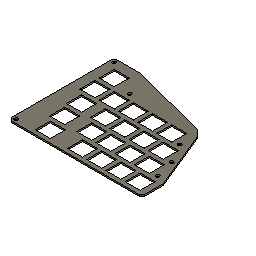
Main Board Plate v2 (Autodesk Fusion 360 design; units mm, degrees)
Autodesk Fusion 360 part; units mm, degrees
note: some values were not read from the file. Set by a fixed rule: which sketch regions a step uses.
(part 1 of 2)
sketch "Sketch1" plane through (0, 0, 0) normal (0, 1, 0) x (1, 0, 0)
  line L0 (0, 0) -> (124, 0)
  line L1 (124, 0) -> (124, 165.5)
  line L2 (124, 165.5) -> (0, 165.5)
  line L3 (0, 165.5) -> (0, 0)
  dimension "d1" = 124
  dimension "d2" = 165.5
  constraint horizontal L0
  constraint vertical L1
  constraint horizontal L2
  constraint vertical L3
  constraint coincident L0.start L3.end
  measures "d1" distance of L0.start L0.end
  measures "d2" distance of L0.start L2.end
extrude "Extrude1" add sketch "Sketch1" along normal blind 1.4
sketch "Sketch2" plane through (0, 1.4, 0) normal (0, 1, 0) x (-1, 0, 0)
  line L0 (0, -165.5) -> (0, 0)
  line L1 (0, 0) -> (-124, 0)
  line L2 (-124, 0) -> (-124, -165.5)
  line L3 (-124, -165.5) -> (0, -165.5)
  line L4 (0, 0) -> (-2.5, 0)
  line L5 (0, 0) -> (0, -2.5)
  line L6 (0, -2.5) -> (-2.5, 0)
  line L7 (-124, 0) -> (-124, -2.5)
  line L8 (-124, 0) -> (-121.5, 0)
  line L9 (-121.5, 0) -> (-124, -2.5)
  line L10 (0, -165.5) -> (0, -163)
  line L11 (0, -165.5) -> (-2.5, -165.5)
  line L12 (-2.5, -165.5) -> (0, -163)
  dimension "d5" = 2.5
  dimension "d6" = 2.5
  dimension "d7" = 2.5
  dimension "d8" = 2.5
  dimension "d9" = 2.5
  constraint coincident L0.end L1.start
  constraint perpendicular L0 L4
  constraint perpendicular L1 L5
  constraint coincident L1.end L2.start
  constraint perpendicular L1 L7
  constraint perpendicular L7 L8
  constraint coincident L0.start L3.end
  constraint coincident L0 L10.end
  constraint perpendicular L1 L10
  constraint perpendicular L10 L11
  measures "d5" distance of L0.end L4.end
  measures "d6" distance of L0.end L5.end
  measures "d7" distance of L1.end L7.end
  measures "d8" distance of L1.end L8.end
  measures "d9" distance of L0.start L11.end
extrude "Extrude2" cut sketch "Sketch2" against normal blind 2 contours L0 L3 L10 L11 L12 | L0 L1 L4 L5 L6 | L1 L2 L7 L8 L9
sketch "Sketch3" plane through (0, 1.4, 0) normal (0, 1, 0) x (-1, 0, 0)
  line L0 (0, -2.5) -> (-2.5, 0)
  line L1 (-2.5, 0) -> (-121.5, 0)
  line L2 (-121.5, 0) -> (-124, -2.5)
  line L3 (-124, -2.5) -> (-124, -165.5)
  line L4 (-124, -165.5) -> (-2.5, -165.5)
  line L5 (-2.5, -165.5) -> (0, -163)
  line L6 (0, -163) -> (0, -2.5)
  line L7 (-2.5, -165.5) -> (0, -165.5)
  line L8 (0, -165.5) -> (-25, -165.5)
  line L9 (0, 0) -> (-96.5, 0)
  line L10 (-96.5, 0) -> (-96.5, -117.5)
  line L11 (0, 0) -> (-102, 0)
  line L12 (-102, 0) -> (-102, -112)
  line L13 (-124, 0) -> (-124, -58)
  line L14 (-25, -165.5) -> (-96.5, -117.5)
  line L15 (-96.5, -117.5) -> (-102, -112)
  line L16 (-102, -112) -> (-124, -58)
  line L17 (-124, -58) -> (-124, -165.5)
  line L18 (-124, -165.5) -> (-25, -165.5)
  dimension "d12" = 25
  dimension "d13" = 96.5
  dimension "d14" = 117.5
  dimension "d15" = 102
  dimension "d16" = 112
  dimension "d17" = 58
  constraint coincident L4.end L5.start
  constraint parallel L4 L7
  constraint parallel L4 L8
  constraint coincident L9.start L11.start
  constraint parallel L1 L9
  constraint perpendicular L1 L10
  constraint parallel L9 L11
  constraint perpendicular L11 L12
  constraint vertical L13
  constraint coincident L3.end L4.start
  measures "d12" distance of L7.end L8.end
  measures "d13" distance of L9.start L9.end
  measures "d14" distance of L9.end L10.end
  measures "d15" distance of L9.start L11.end
  measures "d16" distance of L11.end L12.end
  measures "d17" distance of L13.start L13.end
extrude "Extrude3" cut sketch "Sketch3" against normal blind 5 contours L3 L4 L14 L15 L16 L17 L18
sketch "Sketch4" plane through (0, 1.4, 0) normal (0, 1, 0) x (-1, 0, 0)
  line L0 (-124, -58) -> (-102, -112)
  line L1 (-102, -112) -> (-96.5, -117.5)
  line L2 (-96.5, -117.5) -> (-25, -165.5)
  line L3 (-25, -165.5) -> (-2.5, -165.5)
  line L4 (-2.5, -165.5) -> (0, -163)
  line L5 (0, -163) -> (0, -2.5)
  line L6 (0, -2.5) -> (-2.5, 0)
  line L7 (-2.5, 0) -> (-121.5, 0)
  line L8 (-121.5, 0) -> (-124, -2.5)
  line L9 (-124, -2.5) -> (-124, -58)
  line L10 (0, 0) -> (0, -136.5)
  line L11 (0, -136.5) -> (-30, -136.5)
  line L12 (-25, -165.5) -> (-25, -136.5)
  line L13 (-25, -136.5) -> (-96.5, -117.5)
  dimension "d20" = 136.5
  constraint coincident L10.start origin
  constraint parallel L5 L10
  constraint perpendicular L5 L11
  constraint coincident L2.end L3.start
  constraint coincident L11 L12.end
  constraint perpendicular L11 L12
  constraint coincident L1.end L2.start
  measures "d20" distance of L10.start L10.end
extrude "Extrude4" cut sketch "Sketch4" against normal blind 5 contours L2 L12 L13 | L3 L4 L5 L11 L12
sketch "Sketch5" plane through (0, 1.4, 0) normal (0, 1, 0) x (-1, 0, 0)
  line L0 (-25, -136.5) -> (0, -136.5)
  line L1 (0, -136.5) -> (0, -2.5)
  line L2 (0, -2.5) -> (-2.5, 0)
  line L3 (-2.5, 0) -> (-121.5, 0)
  line L4 (-121.5, 0) -> (-124, -2.5)
  line L5 (-124, -2.5) -> (-124, -58)
  line L6 (-124, -58) -> (-102, -112)
  line L7 (-102, -112) -> (-96.5, -117.5)
  line L8 (-96.5, -117.5) -> (-25, -136.5)
  line L9 (0, -136.5) -> (0, -134)
  line L10 (0, -136.5) -> (-2.5, -136.5)
  line L11 (-2.5, -136.5) -> (0, -134)
  dimension "d23" = 2.5
  constraint coincident L0.end L1.start
  constraint coincident L1 L9.end
  constraint perpendicular L0 L9
  constraint perpendicular L9 L10
  measures "d23" distance of L0.end L10.end
extrude "Extrude5" cut sketch "Sketch5" against normal blind 5 contours L0 L1 L9 L10 L11
sketch "Sketch6" plane through (0, 1.4, 0) normal (0, 1, 0) x (-1, 0, 0)
  line L0 (-2.5, -136.5) -> (0, -134)
  line L1 (0, -134) -> (0, -2.5)
  line L2 (0, -2.5) -> (-2.5, 0)
  line L3 (-2.5, 0) -> (-121.5, 0)
  line L4 (-121.5, 0) -> (-124, -2.5)
  line L5 (-124, -2.5) -> (-124, -58)
  line L6 (-124, -58) -> (-102, -112)
  line L7 (-102, -112) -> (-96.5, -117.5)
  line L8 (-96.5, -117.5) -> (-25, -136.5)
  line L9 (-25, -136.5) -> (-2.5, -136.5)
  line L10 (-2.5, 0) -> (-16, 0)
  line L11 (-16, 0) -> (-16, -120.5)
  line L12 (-11, -116) -> (-21, -116)
  line L13 (-21, -116) -> (-21, -125)
  line L14 (-21, -125) -> (-11, -125)
  line L15 (-11, -125) -> (-11, -116)
  line L16 (-11, -116) -> (-21, -125) construction
  line L17 (-21, -116) -> (-11, -125) construction
  line L18 (-23, -113.5) -> (-9, -113.5)
  line L19 (-9, -113.5) -> (-9, -127.5)
  line L20 (-9, -127.5) -> (-23, -127.5)
  line L21 (-23, -127.5) -> (-23, -113.5)
  line L22 (-23, -113.5) -> (-9, -127.5) construction
  line L23 (-9, -113.5) -> (-23, -127.5) construction
  point P0 (-16, -120.5)
  point P1 (-16, -120.5)
  dimension "d26" = 13.5
  dimension "d27" = 120.5
  dimension "d28" = 14
  dimension "d29" = 14
  constraint coincident L2.end L3.start
  constraint parallel L3 L10
  constraint perpendicular L10 L11
  constraint horizontal L12
  constraint perpendicular L12 L13
  constraint parallel L12 L14
  constraint parallel L13 L15
  constraint coincident L16 P1
  constraint coincident L17 P1
  constraint coincident P1 P0
  constraint horizontal L18
  constraint perpendicular L18 L19
  constraint parallel L18 L20
  constraint parallel L19 L21
  constraint coincident L22 P1
  constraint coincident L23 P1
  measures "d26" distance of L2.end L10.end
  measures "d27" distance of L10.end P1
  measures "d28" distance of L19.end L20.end
  measures "d29" distance of L18.end L19.end
extrude "Extrude6" cut sketch "Sketch6" against normal blind 5 contours L12 L13 L14 L15 | L18 L19 L20 L21
sketch "Sketch7" plane through (0, 1.4, 0) normal (0, 1, 0) x (-1, 0, 0)
  line L0 (-9, -113.5) -> (-9, -127.5)
  line L1 (-9, -127.5) -> (-23, -127.5)
  line L2 (-23, -127.5) -> (-23, -113.5)
  line L3 (-23, -113.5) -> (-9, -113.5)
  line L4 (-2.5, -136.5) -> (0, -134)
  line L5 (0, -134) -> (0, -2.5)
  line L6 (0, -2.5) -> (-2.5, 0)
  line L7 (-2.5, 0) -> (-121.5, 0)
  line L8 (-121.5, 0) -> (-124, -2.5)
  line L9 (-124, -2.5) -> (-124, -58)
  line L10 (-124, -58) -> (-102, -112)
  line L11 (-102, -112) -> (-96.5, -117.5)
  line L12 (-96.5, -117.5) -> (-25, -136.5)
  line L13 (-25, -136.5) -> (-2.5, -136.5)
  line L14 (-16, -120.5) -> (-16, -102.65)
  line L15 (-23, -95.65) -> (-9, -95.65)
  line L16 (-9, -95.65) -> (-9, -109.65)
  line L17 (-9, -109.65) -> (-23, -109.65)
  line L18 (-23, -109.65) -> (-23, -95.65)
  line L19 (-23, -95.65) -> (-9, -109.65) construction
  line L20 (-9, -95.65) -> (-23, -109.65) construction
  line L21 (-16, -102.65) -> (-33.85, -102.65)
  line L22 (-33.85, -102.65) -> (-51.7, -102.65)
  line L23 (-51.7, -102.65) -> (-69.55, -102.65)
  line L24 (-69.55, -102.65) -> (-87.4, -102.65)
  line L25 (-40.85, -95.65) -> (-26.85, -95.65)
  line L26 (-26.85, -95.65) -> (-26.85, -109.65)
  line L27 (-26.85, -109.65) -> (-40.85, -109.65)
  line L28 (-40.85, -109.65) -> (-40.85, -95.65)
  line L29 (-40.85, -95.65) -> (-26.85, -109.65) construction
  line L30 (-26.85, -95.65) -> (-40.85, -109.65) construction
  line L31 (-58.7, -95.65) -> (-44.7, -95.65)
  line L32 (-44.7, -95.65) -> (-44.7, -109.65)
  line L33 (-44.7, -109.65) -> (-58.7, -109.65)
  line L34 (-58.7, -109.65) -> (-58.7, -95.65)
  line L35 (-58.7, -95.65) -> (-44.7, -109.65) construction
  line L36 (-44.7, -95.65) -> (-58.7, -109.65) construction
  line L37 (-76.55, -95.65) -> (-62.55, -95.65)
  line L38 (-62.55, -95.65) -> (-62.55, -109.65)
  line L39 (-62.55, -109.65) -> (-76.55, -109.65)
  line L40 (-76.55, -109.65) -> (-76.55, -95.65)
  line L41 (-76.55, -95.65) -> (-62.55, -109.65) construction
  line L42 (-62.55, -95.65) -> (-76.55, -109.65) construction
  line L43 (-94.4, -95.65) -> (-80.4, -95.65)
  line L44 (-80.4, -95.65) -> (-80.4, -109.65)
  line L45 (-80.4, -109.65) -> (-94.4, -109.65)
  line L46 (-94.4, -109.65) -> (-94.4, -95.65)
  line L47 (-94.4, -95.65) -> (-80.4, -109.65) construction
  line L48 (-80.4, -95.65) -> (-94.4, -109.65) construction
  point P0 (-16, -102.65)
  point P1 (-33.85, -102.65)
  point P2 (-51.7, -102.65)
  point P3 (-69.55, -102.65)
  point P4 (-87.4, -102.65)
  dimension "d32" = 17.85
  dimension "d33" = 14
  dimension "d34" = 14
  dimension "d35" = 17.85
  dimension "d36" = 17.85
  dimension "d37" = 17.85
  dimension "d38" = 17.85
  dimension "d39" = 14
  dimension "d40" = 14
  dimension "d41" = 14
  dimension "d42" = 14
  dimension "d43" = 14
  dimension "d44" = 14
  dimension "d45" = 14
  dimension "d46" = 14
  constraint perpendicular L3 L14
  constraint horizontal L15
  constraint perpendicular L15 L16
  constraint parallel L15 L17
  constraint parallel L16 L18
  constraint coincident L19 P0
  constraint coincident L20 P0
  constraint coincident P0 L14.end
  constraint perpendicular L18 L21
  constraint horizontal L22
  constraint parallel L22 L23
  constraint parallel L23 L24
  constraint horizontal L25
  constraint perpendicular L25 L26
  constraint parallel L25 L27
  constraint parallel L26 L28
  constraint coincident L29 P1
  constraint coincident L30 P1
  constraint coincident P1 L21.end
  constraint horizontal L31
  constraint perpendicular L31 L32
  constraint parallel L31 L33
  constraint parallel L32 L34
  constraint coincident L35 P2
  constraint coincident L36 P2
  constraint coincident P2 L22.end
  constraint horizontal L37
  constraint perpendicular L37 L38
  constraint parallel L37 L39
  constraint parallel L38 L40
  constraint coincident L41 P3
  constraint coincident L42 P3
  constraint coincident P3 L23.end
  constraint horizontal L43
  constraint perpendicular L43 L44
  constraint parallel L43 L45
  constraint parallel L44 L46
  constraint coincident L47 P4
  constraint coincident L48 P4
  constraint coincident P4 L24.end
  measures "d32" distance of L14.start P0
  measures "d33" distance of L16.end L17.end
  measures "d34" distance of L15.end L16.end
  measures "d35" distance of P0 P1
  measures "d36" distance of P1 P2
  measures "d37" distance of P2 P3
  measures "d38" distance of P3 P4
  measures "d39" distance of L26.end L27.end
  measures "d40" distance of L25.end L26.end
  measures "d41" distance of L32.end L33.end
  measures "d42" distance of L31.end L32.end
  measures "d43" distance of L38.end L39.end
  measures "d44" distance of L37.end L38.end
  measures "d45" distance of L44.end L45.end
  measures "d46" distance of L43.end L44.end
extrude "Extrude7" cut sketch "Sketch7" against normal blind 5 contours L14 L17 L18 L21 | L14 L15 L16 L17 L18 L21 | L21 L22 L26 L27 L28 | L21 L22 L25 L26 L28 | L22 L23 L32 L33 L34 | L22 L23 L31 L32 L34 | L23 L24 L38 L39 L40 | L23 L24 L37 L38 L40 | L43 L44 L45 L46
sketch "Sketch8" plane through (0, 1.4, 0) normal (0, 1, 0) x (-1, 0, 0)
  line L0 (-44.7, -95.65) -> (-44.7, -109.65)
  line L1 (-44.7, -109.65) -> (-58.7, -109.65)
  line L2 (-58.7, -109.65) -> (-58.7, -95.65)
  line L3 (-58.7, -95.65) -> (-44.7, -95.65)
  line L4 (-26.85, -95.65) -> (-26.85, -109.65)
  line L5 (-26.85, -109.65) -> (-40.85, -109.65)
  line L6 (-40.85, -109.65) -> (-40.85, -95.65)
  line L7 (-40.85, -95.65) -> (-26.85, -95.65)
  line L8 (-62.55, -95.65) -> (-62.55, -109.65)
  line L9 (-62.55, -109.65) -> (-76.55, -109.65)
  line L10 (-76.55, -109.65) -> (-76.55, -95.65)
  line L11 (-76.55, -95.65) -> (-62.55, -95.65)
  line L12 (-9, -95.65) -> (-9, -109.65)
  line L13 (-9, -109.65) -> (-23, -109.65)
  line L14 (-23, -109.65) -> (-23, -95.65)
  line L15 (-23, -95.65) -> (-9, -95.65)
  line L16 (-80.4, -95.65) -> (-80.4, -109.65)
  line L17 (-80.4, -109.65) -> (-94.4, -109.65)
  line L18 (-94.4, -109.65) -> (-94.4, -95.65)
  line L19 (-94.4, -95.65) -> (-80.4, -95.65)
  line L20 (-9, -113.5) -> (-9, -127.5)
  line L21 (-9, -127.5) -> (-23, -127.5)
  line L22 (-23, -127.5) -> (-23, -113.5)
  line L23 (-23, -113.5) -> (-9, -113.5)
  line L24 (-2.5, -136.5) -> (0, -134)
  line L25 (0, -134) -> (0, -2.5)
  line L26 (0, -2.5) -> (-2.5, 0)
  line L27 (-2.5, 0) -> (-121.5, 0)
  line L28 (-121.5, 0) -> (-124, -2.5)
  line L29 (-124, -2.5) -> (-124, -58)
  line L30 (-124, -58) -> (-102, -112)
  line L31 (-102, -112) -> (-96.5, -117.5)
  line L32 (-96.5, -117.5) -> (-25, -136.5)
  line L33 (-25, -136.5) -> (-2.5, -136.5)
  line L34 (-2.5, 0) -> (-21.325, 0)
  line L35 (-21.325, 0) -> (-21.325, -84.85)
  line L36 (-14.325, -77.85) -> (-28.325, -77.85)
  line L37 (-28.325, -77.85) -> (-28.325, -91.85)
  line L38 (-28.325, -91.85) -> (-14.325, -91.85)
  line L39 (-14.325, -91.85) -> (-14.325, -77.85)
  line L40 (-14.325, -77.85) -> (-28.325, -91.85) construction
  line L41 (-28.325, -77.85) -> (-14.325, -91.85) construction
  line L42 (-21.325, -84.85) -> (-43.75, -84.85)
  line L43 (-36.75, -91.85) -> (-50.75, -91.85)
  line L44 (-50.75, -91.85) -> (-50.75, -77.85)
  line L45 (-50.75, -77.85) -> (-36.75, -77.85)
  line L46 (-36.75, -77.85) -> (-36.75, -91.85)
  line L47 (-36.75, -91.85) -> (-50.75, -77.85) construction
  line L48 (-50.75, -91.85) -> (-36.75, -77.85) construction
  line L49 (-43.75, -84.85) -> (-61.6, -84.85)
  line L50 (-61.6, -84.85) -> (-79.45, -84.85)
  line L51 (-79.45, -84.85) -> (-97.3, -84.85)
  line L52 (-54.6, -91.85) -> (-68.6, -91.85)
  line L53 (-68.6, -91.85) -> (-68.6, -77.85)
  line L54 (-68.6, -77.85) -> (-54.6, -77.85)
  line L55 (-54.6, -77.85) -> (-54.6, -91.85)
  line L56 (-54.6, -91.85) -> (-68.6, -77.85) construction
  line L57 (-68.6, -91.85) -> (-54.6, -77.85) construction
  line L58 (-72.45, -91.85) -> (-86.45, -91.85)
  line L59 (-86.45, -91.85) -> (-86.45, -77.85)
  line L60 (-86.45, -77.85) -> (-72.45, -77.85)
  line L61 (-72.45, -77.85) -> (-72.45, -91.85)
  line L62 (-72.45, -91.85) -> (-86.45, -77.85) construction
  line L63 (-86.45, -91.85) -> (-72.45, -77.85) construction
  line L64 (-90.3, -91.85) -> (-104.3, -91.85)
  line L65 (-104.3, -91.85) -> (-104.3, -77.85)
  line L66 (-104.3, -77.85) -> (-90.3, -77.85)
  line L67 (-90.3, -77.85) -> (-90.3, -91.85)
  line L68 (-90.3, -91.85) -> (-104.3, -77.85) construction
  line L69 (-104.3, -91.85) -> (-90.3, -77.85) construction
  point P0 (-21.325, -84.85)
  point P1 (-43.75, -84.85)
  point P2 (-61.6, -84.85)
  point P3 (-79.45, -84.85)
  point P4 (-97.3, -84.85)
  dimension "d49" = 18.825
  dimension "d50" = 84.85
  dimension "d51" = 14
  dimension "d52" = 14
  dimension "d53" = 22.425
  dimension "d54" = 14
  dimension "d55" = 14
  dimension "d56" = 17.85
  dimension "d57" = 17.85
  dimension "d58" = 17.85
  dimension "d59" = 14
  dimension "d60" = 14
  dimension "d61" = 14
  dimension "d62" = 14
  dimension "d63" = 14
  dimension "d64" = 14
  constraint coincident L26.end L27.start
  constraint parallel L27 L34
  constraint perpendicular L34 L35
  constraint horizontal L36
  constraint perpendicular L36 L37
  constraint parallel L36 L38
  constraint parallel L37 L39
  constraint coincident L40 P0
  constraint coincident L41 P0
  constraint coincident P0 L35.end
  constraint perpendicular L37 L42
  constraint horizontal L43
  constraint perpendicular L43 L44
  constraint parallel L43 L45
  constraint parallel L44 L46
  constraint coincident L47 P1
  constraint coincident L48 P1
  constraint coincident P1 L42.end
  constraint perpendicular L44 L49
  constraint horizontal L50
  constraint parallel L50 L51
  constraint horizontal L52
  constraint perpendicular L52 L53
  constraint parallel L52 L54
  constraint parallel L53 L55
  constraint coincident L56 P2
  constraint coincident L57 P2
  constraint coincident P2 L49.end
  constraint horizontal L58
  constraint perpendicular L58 L59
  constraint parallel L58 L60
  constraint parallel L59 L61
  constraint coincident L62 P3
  constraint coincident L63 P3
  constraint coincident P3 L50.end
  constraint horizontal L64
  constraint perpendicular L64 L65
  constraint parallel L64 L66
  constraint parallel L65 L67
  constraint coincident L68 P4
  constraint coincident L69 P4
  constraint coincident P4 L51.end
  measures "d49" distance of L26.end L34.end
  measures "d50" distance of L34.end P0
  measures "d51" distance of L37.end L38.end
  measures "d52" distance of L36.end L37.end
  measures "d53" distance of P0 P1
  measures "d54" distance of L44.end L45.end
  measures "d55" distance of L43.end L44.end
  measures "d56" distance of P1 P2
  measures "d57" distance of P2 P3
  measures "d58" distance of P3 P4
  measures "d59" distance of L53.end L54.end
  measures "d60" distance of L52.end L53.end
  measures "d61" distance of L59.end L60.end
  measures "d62" distance of L58.end L59.end
  measures "d63" distance of L65.end L66.end
  measures "d64" distance of L64.end L65.end
extrude "Extrude8" cut sketch "Sketch8" against normal blind 5 contours L35 L36 L37 L38 L39 L42 | L35 L36 L37 L42 | L42 L43 L44 L46 L49 | L42 L44 L45 L46 L49 | L49 L50 L52 L53 L55 | L49 L50 L53 L54 L55 | L50 L51 L58 L59 L61 | L50 L51 L59 L60 L61 | L64 L65 L66 L67
sketch "Sketch9" plane through (0, 1.4, 0) normal (0, 1, 0) x (-1, 0, 0)
  line L0 (-68.6, -91.85) -> (-68.6, -77.85)
  line L1 (-68.6, -77.85) -> (-54.6, -77.85)
  line L2 (-54.6, -77.85) -> (-54.6, -91.85)
  line L3 (-54.6, -91.85) -> (-68.6, -91.85)
  line L4 (-50.75, -91.85) -> (-50.75, -77.85)
  line L5 (-50.75, -77.85) -> (-36.75, -77.85)
  line L6 (-36.75, -77.85) -> (-36.75, -91.85)
  line L7 (-36.75, -91.85) -> (-50.75, -91.85)
  line L8 (-86.45, -91.85) -> (-86.45, -77.85)
  line L9 (-86.45, -77.85) -> (-72.45, -77.85)
  line L10 (-72.45, -77.85) -> (-72.45, -91.85)
  line L11 (-72.45, -91.85) -> (-86.45, -91.85)
  line L12 (-28.325, -77.85) -> (-14.325, -77.85)
  line L13 (-14.325, -77.85) -> (-14.325, -91.85)
  line L14 (-14.325, -91.85) -> (-28.325, -91.85)
  line L15 (-28.325, -91.85) -> (-28.325, -77.85)
  line L16 (-104.3, -91.85) -> (-104.3, -77.85)
  line L17 (-104.3, -77.85) -> (-90.3, -77.85)
  line L18 (-90.3, -77.85) -> (-90.3, -91.85)
  line L19 (-90.3, -91.85) -> (-104.3, -91.85)
  line L20 (-44.7, -95.65) -> (-44.7, -109.65)
  line L21 (-44.7, -109.65) -> (-58.7, -109.65)
  line L22 (-58.7, -109.65) -> (-58.7, -95.65)
  line L23 (-58.7, -95.65) -> (-44.7, -95.65)
  line L24 (-26.85, -95.65) -> (-26.85, -109.65)
  line L25 (-26.85, -109.65) -> (-40.85, -109.65)
  line L26 (-40.85, -109.65) -> (-40.85, -95.65)
  line L27 (-40.85, -95.65) -> (-26.85, -95.65)
  line L28 (-62.55, -95.65) -> (-62.55, -109.65)
  line L29 (-62.55, -109.65) -> (-76.55, -109.65)
  line L30 (-76.55, -109.65) -> (-76.55, -95.65)
  line L31 (-76.55, -95.65) -> (-62.55, -95.65)
  line L32 (-9, -95.65) -> (-9, -109.65)
  line L33 (-9, -109.65) -> (-23, -109.65)
  line L34 (-23, -109.65) -> (-23, -95.65)
  line L35 (-23, -95.65) -> (-9, -95.65)
  line L36 (-80.4, -95.65) -> (-80.4, -109.65)
  line L37 (-80.4, -109.65) -> (-94.4, -109.65)
  line L38 (-94.4, -109.65) -> (-94.4, -95.65)
  line L39 (-94.4, -95.65) -> (-80.4, -95.65)
  line L40 (-9, -113.5) -> (-9, -127.5)
  line L41 (-9, -127.5) -> (-23, -127.5)
  line L42 (-23, -127.5) -> (-23, -113.5)
  line L43 (-23, -113.5) -> (-9, -113.5)
  line L44 (-2.5, -136.5) -> (0, -134)
  line L45 (0, -134) -> (0, -2.5)
  line L46 (0, -2.5) -> (-2.5, 0)
  line L47 (-2.5, 0) -> (-121.5, 0)
  line L48 (-121.5, 0) -> (-124, -2.5)
  line L49 (-124, -2.5) -> (-124, -58)
  line L50 (-124, -58) -> (-102, -112)
  line L51 (-102, -112) -> (-96.5, -117.5)
  line L52 (-96.5, -117.5) -> (-25, -136.5)
  line L53 (-25, -136.5) -> (-2.5, -136.5)
  line L54 (-19.35, -102.65) -> (-19.35, -66.95)
  line L55 (-19.35, -66.95) -> (-26.675, -66.95)
  line L56 (-33.675, -73.95) -> (-19.675, -73.95)
  line L57 (-19.675, -73.95) -> (-19.675, -59.95)
  line L58 (-19.675, -59.95) -> (-33.675, -59.95)
  line L59 (-33.675, -59.95) -> (-33.675, -73.95)
  line L60 (-33.675, -73.95) -> (-19.675, -59.95) construction
  line L61 (-19.675, -73.95) -> (-33.675, -59.95) construction
  line L62 (-26.675, -66.95) -> (-51.85, -66.95)
  line L63 (-58.85, -59.95) -> (-44.85, -59.95)
  line L64 (-44.85, -59.95) -> (-44.85, -73.95)
  line L65 (-44.85, -73.95) -> (-58.85, -73.95)
  line L66 (-58.85, -73.95) -> (-58.85, -59.95)
  line L67 (-58.85, -59.95) -> (-44.85, -73.95) construction
  line L68 (-44.85, -59.95) -> (-58.85, -73.95) construction
  line L69 (-51.85, -66.95) -> (-69.7, -66.95)
  line L70 (-69.7, -66.95) -> (-87.55, -66.95)
  line L71 (-87.55, -66.95) -> (-105.4, -66.95)
  line L72 (-76.7, -73.95) -> (-62.7, -73.95)
  line L73 (-62.7, -73.95) -> (-62.7, -59.95)
  line L74 (-62.7, -59.95) -> (-76.7, -59.95)
  line L75 (-76.7, -59.95) -> (-76.7, -73.95)
  line L76 (-76.7, -73.95) -> (-62.7, -59.95) construction
  line L77 (-62.7, -73.95) -> (-76.7, -59.95) construction
  line L78 (-94.55, -73.95) -> (-80.55, -73.95)
  line L79 (-80.55, -73.95) -> (-80.55, -59.95)
  line L80 (-80.55, -59.95) -> (-94.55, -59.95)
  line L81 (-94.55, -59.95) -> (-94.55, -73.95)
  line L82 (-94.55, -73.95) -> (-80.55, -59.95) construction
  line L83 (-80.55, -73.95) -> (-94.55, -59.95) construction
  line L84 (-112.4, -59.95) -> (-98.4, -59.95)
  line L85 (-98.4, -59.95) -> (-98.4, -73.95)
  line L86 (-98.4, -73.95) -> (-112.4, -73.95)
  line L87 (-112.4, -73.95) -> (-112.4, -59.95)
  line L88 (-112.4, -59.95) -> (-98.4, -73.95) construction
  line L89 (-98.4, -59.95) -> (-112.4, -73.95) construction
  point P0 (-26.675, -66.95)
  point P1 (-51.85, -66.95)
  point P2 (-69.7, -66.95)
  point P3 (-87.55, -66.95)
  point P4 (-105.4, -66.95)
  dimension "d67" = 35.7
  dimension "d68" = 7.325
  dimension "d69" = 14
  dimension "d70" = 14
  dimension "d71" = 25.175
  dimension "d72" = 14
  dimension "d73" = 14
  dimension "d74" = 17.85
  dimension "d75" = 17.85
  dimension "d76" = 17.85
  dimension "d77" = 14
  dimension "d78" = 14
  dimension "d79" = 14
  dimension "d80" = 14
  dimension "d81" = 14
  dimension "d82" = 14
  constraint perpendicular L14 L54
  constraint perpendicular L54 L55
  constraint horizontal L56
  constraint perpendicular L56 L57
  constraint parallel L56 L58
  constraint parallel L57 L59
  constraint coincident L60 P0
  constraint coincident L61 P0
  constraint coincident P0 L55.end
  constraint perpendicular L59 L62
  constraint horizontal L63
  constraint perpendicular L63 L64
  constraint parallel L63 L65
  constraint parallel L64 L66
  constraint coincident L67 P1
  constraint coincident L68 P1
  constraint coincident P1 L62.end
  constraint perpendicular L66 L69
  constraint parallel L69 L70
  constraint parallel L70 L71
  constraint horizontal L72
  constraint perpendicular L72 L73
  constraint parallel L72 L74
  constraint parallel L73 L75
  constraint coincident L76 P2
  constraint coincident L77 P2
  constraint coincident P2 L69.end
  constraint horizontal L78
  constraint perpendicular L78 L79
  constraint parallel L78 L80
  constraint parallel L79 L81
  constraint coincident L82 P3
  constraint coincident L83 P3
  constraint coincident P3 L70.end
  constraint horizontal L84
  constraint perpendicular L84 L85
  constraint parallel L84 L86
  constraint parallel L85 L87
  constraint coincident L88 P4
  constraint coincident L89 P4
  constraint coincident P4 L71.end
  measures "d67" distance of L54.start L54.end
  measures "d68" distance of L54.end P0
  measures "d69" distance of L57.end L58.end
  measures "d70" distance of L56.end L57.end
  measures "d71" distance of P0 P1
  measures "d72" distance of L64.end L65.end
  measures "d73" distance of L63.end L64.end
  measures "d74" distance of P1 P2
  measures "d75" distance of P2 P3
  measures "d76" distance of P3 P4
  measures "d77" distance of L73.end L74.end
  measures "d78" distance of L72.end L73.end
  measures "d79" distance of L79.end L80.end
  measures "d80" distance of L78.end L79.end
  measures "d81" distance of L85.end L86.end
  measures "d82" distance of L84.end L85.end
extrude "Extrude9" cut sketch "Sketch9" against normal blind 5 contours L55 L56 L57 L59 L62 | L55 L57 L58 L59 L62 | L62 L64 L65 L66 L69 | L62 L63 L64 L66 L69 | L69 L70 L72 L73 L75 | L69 L70 L73 L74 L75 | L70 L71 L78 L79 L81 | L70 L71 L79 L80 L81 | L84 L85 L86 L87
sketch "Sketch10" plane through (0, 1.4, 0) normal (0, 1, 0) x (-1, 0, 0)
  line L0 (-62.7, -73.95) -> (-76.7, -73.95)
  line L1 (-76.7, -73.95) -> (-76.7, -59.95)
  line L2 (-76.7, -59.95) -> (-62.7, -59.95)
  line L3 (-62.7, -59.95) -> (-62.7, -73.95)
  line L4 (-44.85, -59.95) -> (-44.85, -73.95)
  line L5 (-44.85, -73.95) -> (-58.85, -73.95)
  line L6 (-58.85, -73.95) -> (-58.85, -59.95)
  line L7 (-58.85, -59.95) -> (-44.85, -59.95)
  line L8 (-80.55, -73.95) -> (-94.55, -73.95)
  line L9 (-94.55, -73.95) -> (-94.55, -59.95)
  line L10 (-94.55, -59.95) -> (-80.55, -59.95)
  line L11 (-80.55, -59.95) -> (-80.55, -73.95)
  line L12 (-19.675, -73.95) -> (-33.675, -73.95)
  line L13 (-33.675, -73.95) -> (-33.675, -59.95)
  line L14 (-33.675, -59.95) -> (-19.675, -59.95)
  line L15 (-19.675, -59.95) -> (-19.675, -73.95)
  line L16 (-98.4, -59.95) -> (-98.4, -73.95)
  line L17 (-98.4, -73.95) -> (-112.4, -73.95)
  line L18 (-112.4, -73.95) -> (-112.4, -59.95)
  line L19 (-112.4, -59.95) -> (-98.4, -59.95)
  line L20 (-68.6, -91.85) -> (-68.6, -77.85)
  line L21 (-68.6, -77.85) -> (-54.6, -77.85)
  line L22 (-54.6, -77.85) -> (-54.6, -91.85)
  line L23 (-54.6, -91.85) -> (-68.6, -91.85)
  line L24 (-50.75, -91.85) -> (-50.75, -77.85)
  line L25 (-50.75, -77.85) -> (-36.75, -77.85)
  line L26 (-36.75, -77.85) -> (-36.75, -91.85)
  line L27 (-36.75, -91.85) -> (-50.75, -91.85)
  line L28 (-86.45, -91.85) -> (-86.45, -77.85)
  line L29 (-86.45, -77.85) -> (-72.45, -77.85)
  line L30 (-72.45, -77.85) -> (-72.45, -91.85)
  line L31 (-72.45, -91.85) -> (-86.45, -91.85)
  line L32 (-28.325, -77.85) -> (-14.325, -77.85)
  line L33 (-14.325, -77.85) -> (-14.325, -91.85)
  line L34 (-14.325, -91.85) -> (-28.325, -91.85)
  line L35 (-28.325, -91.85) -> (-28.325, -77.85)
  line L36 (-104.3, -91.85) -> (-104.3, -77.85)
  line L37 (-104.3, -77.85) -> (-90.3, -77.85)
  line L38 (-90.3, -77.85) -> (-90.3, -91.85)
  line L39 (-90.3, -91.85) -> (-104.3, -91.85)
  line L40 (-44.7, -95.65) -> (-44.7, -109.65)
  line L41 (-44.7, -109.65) -> (-58.7, -109.65)
  line L42 (-58.7, -109.65) -> (-58.7, -95.65)
  line L43 (-58.7, -95.65) -> (-44.7, -95.65)
  line L44 (-26.85, -95.65) -> (-26.85, -109.65)
  line L45 (-26.85, -109.65) -> (-40.85, -109.65)
  line L46 (-40.85, -109.65) -> (-40.85, -95.65)
  line L47 (-40.85, -95.65) -> (-26.85, -95.65)
  line L48 (-62.55, -95.65) -> (-62.55, -109.65)
  line L49 (-62.55, -109.65) -> (-76.55, -109.65)
  line L50 (-76.55, -109.65) -> (-76.55, -95.65)
  line L51 (-76.55, -95.65) -> (-62.55, -95.65)
  line L52 (-9, -95.65) -> (-9, -109.65)
  line L53 (-9, -109.65) -> (-23, -109.65)
  line L54 (-23, -109.65) -> (-23, -95.65)
  line L55 (-23, -95.65) -> (-9, -95.65)
  line L56 (-80.4, -95.65) -> (-80.4, -109.65)
  line L57 (-80.4, -109.65) -> (-94.4, -109.65)
  line L58 (-94.4, -109.65) -> (-94.4, -95.65)
  line L59 (-94.4, -95.65) -> (-80.4, -95.65)
  line L60 (-9, -113.5) -> (-9, -127.5)
  line L61 (-9, -127.5) -> (-23, -127.5)
  line L62 (-23, -127.5) -> (-23, -113.5)
  line L63 (-23, -113.5) -> (-9, -113.5)
  line L64 (-2.5, -136.5) -> (0, -134)
  line L65 (0, -134) -> (0, -2.5)
  line L66 (0, -2.5) -> (-2.5, 0)
  line L67 (-2.5, 0) -> (-121.5, 0)
  line L68 (-121.5, 0) -> (-124, -2.5)
  line L69 (-124, -2.5) -> (-124, -58)
  line L70 (-124, -58) -> (-102, -112)
  line L71 (-102, -112) -> (-96.5, -117.5)
  line L72 (-96.5, -117.5) -> (-25, -136.5)
  line L73 (-25, -136.5) -> (-2.5, -136.5)
  line L74 (-16, -120.5) -> (-16, -49.1)
  line L75 (-16, -49.1) -> (-28.075, -49.1)
  line L76 (-35.075, -56.1) -> (-21.075, -56.1)
  line L77 (-21.075, -56.1) -> (-21.075, -42.1)
  line L78 (-21.075, -42.1) -> (-35.075, -42.1)
  line L79 (-35.075, -42.1) -> (-35.075, -56.1)
  line L80 (-35.075, -56.1) -> (-21.075, -42.1) construction
  line L81 (-21.075, -56.1) -> (-35.075, -42.1) construction
  line L82 (-28.075, -49.1) -> (-58, -49.1)
  line L83 (-58, -49.1) -> (-75.85, -49.1)
  line L84 (-75.85, -49.1) -> (-93.7, -49.1)
  line L85 (-93.7, -49.1) -> (-111.55, -49.1)
  line L86 (-65, -56.1) -> (-51, -56.1)
  line L87 (-51, -56.1) -> (-51, -42.1)
  line L88 (-51, -42.1) -> (-65, -42.1)
  line L89 (-65, -42.1) -> (-65, -56.1)
  line L90 (-65, -56.1) -> (-51, -42.1) construction
  line L91 (-51, -56.1) -> (-65, -42.1) construction
  line L92 (-82.85, -56.1) -> (-68.85, -56.1)
  line L93 (-68.85, -56.1) -> (-68.85, -42.1)
  line L94 (-68.85, -42.1) -> (-82.85, -42.1)
  line L95 (-82.85, -42.1) -> (-82.85, -56.1)
  line L96 (-82.85, -56.1) -> (-68.85, -42.1) construction
  line L97 (-68.85, -56.1) -> (-82.85, -42.1) construction
  line L98 (-100.7, -56.1) -> (-86.7, -56.1)
  line L99 (-86.7, -56.1) -> (-86.7, -42.1)
  line L100 (-86.7, -42.1) -> (-100.7, -42.1)
  line L101 (-100.7, -42.1) -> (-100.7, -56.1)
  line L102 (-100.7, -56.1) -> (-86.7, -42.1) construction
  line L103 (-86.7, -56.1) -> (-100.7, -42.1) construction
  line L104 (-118.55, -56.1) -> (-104.55, -56.1)
  line L105 (-104.55, -56.1) -> (-104.55, -42.1)
  line L106 (-104.55, -42.1) -> (-118.55, -42.1)
  line L107 (-118.55, -42.1) -> (-118.55, -56.1)
  line L108 (-118.55, -56.1) -> (-104.55, -42.1) construction
  line L109 (-104.55, -56.1) -> (-118.55, -42.1) construction
  point P0 (-28.075, -49.1)
  point P1 (-58, -49.1)
  point P2 (-75.85, -49.1)
  point P3 (-93.7, -49.1)
  point P4 (-111.55, -49.1)
  dimension "d85" = 71.4
  dimension "d86" = 12.075
  dimension "d87" = 14
  dimension "d88" = 14
  dimension "d89" = 29.925
  dimension "d90" = 17.85
  dimension "d91" = 17.85
  dimension "d92" = 17.85
  dimension "d93" = 14
  dimension "d94" = 14
  dimension "d95" = 14
  dimension "d96" = 14
  dimension "d97" = 14
  dimension "d98" = 14
  dimension "d99" = 14
  dimension "d100" = 14
  constraint perpendicular L34 L74
  constraint perpendicular L74 L75
  constraint horizontal L76
  constraint perpendicular L76 L77
  constraint parallel L76 L78
  constraint parallel L77 L79
  constraint coincident L80 P0
  constraint coincident L81 P0
  constraint coincident P0 L75.end
  constraint perpendicular L79 L82
  constraint parallel L82 L83
  constraint horizontal L84
  constraint parallel L84 L85
  constraint horizontal L86
  constraint perpendicular L86 L87
  constraint parallel L86 L88
  constraint parallel L87 L89
  constraint coincident L90 P1
  constraint coincident L91 P1
  constraint coincident P1 L82.end
  constraint horizontal L92
  constraint perpendicular L92 L93
  constraint parallel L92 L94
  constraint parallel L93 L95
  constraint coincident L96 P2
  constraint coincident L97 P2
  constraint coincident P2 L83.end
  constraint horizontal L98
  constraint perpendicular L98 L99
  constraint parallel L98 L100
  constraint parallel L99 L101
  constraint coincident L102 P3
  constraint coincident L103 P3
  constraint coincident P3 L84.end
  constraint horizontal L104
  constraint perpendicular L104 L105
  constraint parallel L104 L106
  constraint parallel L105 L107
  constraint coincident L108 P4
  constraint coincident L109 P4
  constraint coincident P4 L85.end
  measures "d85" distance of L74.start L74.end
  measures "d86" distance of L74.end P0
  measures "d87" distance of L77.end L78.end
  measures "d88" distance of L76.end L77.end
  measures "d89" distance of P0 P1
  measures "d90" distance of P1 P2
  measures "d91" distance of P2 P3
  measures "d92" distance of P3 P4
  measures "d93" distance of L87.end L88.end
  measures "d94" distance of L86.end L87.end
  measures "d95" distance of L93.end L94.end
  measures "d96" distance of L92.end L93.end
  measures "d97" distance of L99.end L100.end
  measures "d98" distance of L98.end L99.end
  measures "d99" distance of L105.end L106.end
  measures "d100" distance of L104.end L105.end
extrude "Extrude10" cut sketch "Sketch10" against normal blind 5 contours L75 L76 L77 L79 L82 | L75 L77 L78 L79 L82 | L82 L83 L86 L87 L89 | L82 L83 L87 L88 L89 | L83 L84 L92 L93 L95 | L83 L84 L93 L94 L95 | L84 L85 L98 L99 L101 | L84 L85 L99 L100 L101 | L104 L105 L106 L107
sketch "Sketch11" plane through (0, 1.4, 0) normal (0, 1, 0) x (-1, 0, 0)
  line L0 (-68.85, -56.1) -> (-82.85, -56.1)
  line L1 (-82.85, -56.1) -> (-82.85, -42.1)
  line L2 (-82.85, -42.1) -> (-68.85, -42.1)
  line L3 (-68.85, -42.1) -> (-68.85, -56.1)
  line L4 (-51, -56.1) -> (-65, -56.1)
  line L5 (-65, -56.1) -> (-65, -42.1)
  line L6 (-65, -42.1) -> (-51, -42.1)
  line L7 (-51, -42.1) -> (-51, -56.1)
  line L8 (-86.7, -56.1) -> (-100.7, -56.1)
  line L9 (-100.7, -56.1) -> (-100.7, -42.1)
  line L10 (-100.7, -42.1) -> (-86.7, -42.1)
  line L11 (-86.7, -42.1) -> (-86.7, -56.1)
  line L12 (-21.075, -56.1) -> (-35.075, -56.1)
  line L13 (-35.075, -56.1) -> (-35.075, -42.1)
  line L14 (-35.075, -42.1) -> (-21.075, -42.1)
  line L15 (-21.075, -42.1) -> (-21.075, -56.1)
  line L16 (-104.55, -56.1) -> (-118.55, -56.1)
  line L17 (-118.55, -56.1) -> (-118.55, -42.1)
  line L18 (-118.55, -42.1) -> (-104.55, -42.1)
  line L19 (-104.55, -42.1) -> (-104.55, -56.1)
  line L20 (-62.7, -73.95) -> (-76.7, -73.95)
  line L21 (-76.7, -73.95) -> (-76.7, -59.95)
  line L22 (-76.7, -59.95) -> (-62.7, -59.95)
  line L23 (-62.7, -59.95) -> (-62.7, -73.95)
  line L24 (-44.85, -59.95) -> (-44.85, -73.95)
  line L25 (-44.85, -73.95) -> (-58.85, -73.95)
  line L26 (-58.85, -73.95) -> (-58.85, -59.95)
  line L27 (-58.85, -59.95) -> (-44.85, -59.95)
  line L28 (-80.55, -73.95) -> (-94.55, -73.95)
  line L29 (-94.55, -73.95) -> (-94.55, -59.95)
  line L30 (-94.55, -59.95) -> (-80.55, -59.95)
  line L31 (-80.55, -59.95) -> (-80.55, -73.95)
  line L32 (-19.675, -73.95) -> (-33.675, -73.95)
  line L33 (-33.675, -73.95) -> (-33.675, -59.95)
  line L34 (-33.675, -59.95) -> (-19.675, -59.95)
  line L35 (-19.675, -59.95) -> (-19.675, -73.95)
  line L36 (-98.4, -59.95) -> (-98.4, -73.95)
  line L37 (-98.4, -73.95) -> (-112.4, -73.95)
  line L38 (-112.4, -73.95) -> (-112.4, -59.95)
  line L39 (-112.4, -59.95) -> (-98.4, -59.95)
  line L40 (-68.6, -91.85) -> (-68.6, -77.85)
  line L41 (-68.6, -77.85) -> (-54.6, -77.85)
  line L42 (-54.6, -77.85) -> (-54.6, -91.85)
  line L43 (-54.6, -91.85) -> (-68.6, -91.85)
  line L44 (-50.75, -91.85) -> (-50.75, -77.85)
  line L45 (-50.75, -77.85) -> (-36.75, -77.85)
  line L46 (-36.75, -77.85) -> (-36.75, -91.85)
  line L47 (-36.75, -91.85) -> (-50.75, -91.85)
  line L48 (-86.45, -91.85) -> (-86.45, -77.85)
  line L49 (-86.45, -77.85) -> (-72.45, -77.85)
  line L50 (-72.45, -77.85) -> (-72.45, -91.85)
  line L51 (-72.45, -91.85) -> (-86.45, -91.85)
  line L52 (-28.325, -77.85) -> (-14.325, -77.85)
  line L53 (-14.325, -77.85) -> (-14.325, -91.85)
  line L54 (-14.325, -91.85) -> (-28.325, -91.85)
  line L55 (-28.325, -91.85) -> (-28.325, -77.85)
  line L56 (-104.3, -91.85) -> (-104.3, -77.85)
  line L57 (-104.3, -77.85) -> (-90.3, -77.85)
  line L58 (-90.3, -77.85) -> (-90.3, -91.85)
  line L59 (-90.3, -91.85) -> (-104.3, -91.85)
  line L60 (-44.7, -95.65) -> (-44.7, -109.65)
  line L61 (-44.7, -109.65) -> (-58.7, -109.65)
  line L62 (-58.7, -109.65) -> (-58.7, -95.65)
  line L63 (-58.7, -95.65) -> (-44.7, -95.65)
  line L64 (-26.85, -95.65) -> (-26.85, -109.65)
  line L65 (-26.85, -109.65) -> (-40.85, -109.65)
  line L66 (-40.85, -109.65) -> (-40.85, -95.65)
  line L67 (-40.85, -95.65) -> (-26.85, -95.65)
  line L68 (-62.55, -95.65) -> (-62.55, -109.65)
  line L69 (-62.55, -109.65) -> (-76.55, -109.65)
  line L70 (-76.55, -109.65) -> (-76.55, -95.65)
  line L71 (-76.55, -95.65) -> (-62.55, -95.65)
  line L72 (-9, -95.65) -> (-9, -109.65)
  line L73 (-9, -109.65) -> (-23, -109.65)
  line L74 (-23, -109.65) -> (-23, -95.65)
  line L75 (-23, -95.65) -> (-9, -95.65)
  line L76 (-80.4, -95.65) -> (-80.4, -109.65)
  line L77 (-80.4, -109.65) -> (-94.4, -109.65)
  line L78 (-94.4, -109.65) -> (-94.4, -95.65)
  line L79 (-94.4, -95.65) -> (-80.4, -95.65)
  line L80 (-9, -113.5) -> (-9, -127.5)
  line L81 (-9, -127.5) -> (-23, -127.5)
  line L82 (-23, -127.5) -> (-23, -113.5)
  line L83 (-23, -113.5) -> (-9, -113.5)
  line L84 (-2.5, -136.5) -> (0, -134)
  line L85 (0, -134) -> (0, -2.5)
  line L86 (0, -2.5) -> (-2.5, 0)
  line L87 (-2.5, 0) -> (-121.5, 0)
  line L88 (-121.5, 0) -> (-124, -2.5)
  line L89 (-124, -2.5) -> (-124, -58)
  line L90 (-124, -58) -> (-102, -112)
  line L91 (-102, -112) -> (-96.5, -117.5)
  line L92 (-96.5, -117.5) -> (-25, -136.5)
  line L93 (-25, -136.5) -> (-2.5, -136.5)
  line L94 (-58.8827, -42.1) -> (-58.8827, -38.25)
  line L95 (-58.8827, -38.25) -> (-124, -38.25)
  line L96 (-58.8827, -38.25) -> (0, -38.25)
  dimension "d103" = 3.85
  constraint coincident L6 L94.start
  constraint perpendicular L6 L94
  constraint perpendicular L94 L95
  constraint coincident L85 L96.end
  constraint perpendicular L85 L96
  measures "d103" distance of L94.start L94.end
extrude "Extrude11" cut sketch "Sketch11" against normal blind 5 contours L85 L86 L87 L88 L89 L95 L96
sketch "Sketch12" plane through (0, 1.4, 0) normal (0, 1, 0) x (-1, 0, 0)
  line L0 (0, -38.25) -> (-124, -38.25)
  line L1 (-124, -38.25) -> (-124, -58)
  line L2 (-124, -58) -> (-102, -112)
  line L3 (-102, -112) -> (-96.5, -117.5)
  line L4 (-96.5, -117.5) -> (-25, -136.5)
  line L5 (-25, -136.5) -> (-2.5, -136.5)
  line L6 (-2.5, -136.5) -> (0, -134)
  line L7 (0, -134) -> (0, -38.25)
  line L8 (-68.85, -56.1) -> (-82.85, -56.1)
  line L9 (-82.85, -56.1) -> (-82.85, -42.1)
  line L10 (-82.85, -42.1) -> (-68.85, -42.1)
  line L11 (-68.85, -42.1) -> (-68.85, -56.1)
  line L12 (-51, -56.1) -> (-65, -56.1)
  line L13 (-65, -56.1) -> (-65, -42.1)
  line L14 (-65, -42.1) -> (-51, -42.1)
  line L15 (-51, -42.1) -> (-51, -56.1)
  line L16 (-86.7, -56.1) -> (-100.7, -56.1)
  line L17 (-100.7, -56.1) -> (-100.7, -42.1)
  line L18 (-100.7, -42.1) -> (-86.7, -42.1)
  line L19 (-86.7, -42.1) -> (-86.7, -56.1)
  line L20 (-21.075, -56.1) -> (-35.075, -56.1)
  line L21 (-35.075, -56.1) -> (-35.075, -42.1)
  line L22 (-35.075, -42.1) -> (-21.075, -42.1)
  line L23 (-21.075, -42.1) -> (-21.075, -56.1)
  line L24 (-104.55, -56.1) -> (-118.55, -56.1)
  line L25 (-118.55, -56.1) -> (-118.55, -42.1)
  line L26 (-118.55, -42.1) -> (-104.55, -42.1)
  line L27 (-104.55, -42.1) -> (-104.55, -56.1)
  line L28 (-62.7, -73.95) -> (-76.7, -73.95)
  line L29 (-76.7, -73.95) -> (-76.7, -59.95)
  line L30 (-76.7, -59.95) -> (-62.7, -59.95)
  line L31 (-62.7, -59.95) -> (-62.7, -73.95)
  line L32 (-44.85, -59.95) -> (-44.85, -73.95)
  line L33 (-44.85, -73.95) -> (-58.85, -73.95)
  line L34 (-58.85, -73.95) -> (-58.85, -59.95)
  line L35 (-58.85, -59.95) -> (-44.85, -59.95)
  line L36 (-80.55, -73.95) -> (-94.55, -73.95)
  line L37 (-94.55, -73.95) -> (-94.55, -59.95)
  line L38 (-94.55, -59.95) -> (-80.55, -59.95)
  line L39 (-80.55, -59.95) -> (-80.55, -73.95)
  line L40 (-19.675, -73.95) -> (-33.675, -73.95)
  line L41 (-33.675, -73.95) -> (-33.675, -59.95)
  line L42 (-33.675, -59.95) -> (-19.675, -59.95)
  line L43 (-19.675, -59.95) -> (-19.675, -73.95)
  line L44 (-98.4, -59.95) -> (-98.4, -73.95)
  line L45 (-98.4, -73.95) -> (-112.4, -73.95)
  line L46 (-112.4, -73.95) -> (-112.4, -59.95)
  line L47 (-112.4, -59.95) -> (-98.4, -59.95)
  line L48 (-68.6, -91.85) -> (-68.6, -77.85)
  line L49 (-68.6, -77.85) -> (-54.6, -77.85)
  line L50 (-54.6, -77.85) -> (-54.6, -91.85)
  line L51 (-54.6, -91.85) -> (-68.6, -91.85)
  line L52 (-50.75, -91.85) -> (-50.75, -77.85)
  line L53 (-50.75, -77.85) -> (-36.75, -77.85)
  line L54 (-36.75, -77.85) -> (-36.75, -91.85)
  line L55 (-36.75, -91.85) -> (-50.75, -91.85)
  line L56 (-86.45, -91.85) -> (-86.45, -77.85)
  line L57 (-86.45, -77.85) -> (-72.45, -77.85)
  line L58 (-72.45, -77.85) -> (-72.45, -91.85)
  line L59 (-72.45, -91.85) -> (-86.45, -91.85)
  line L60 (-28.325, -77.85) -> (-14.325, -77.85)
  line L61 (-14.325, -77.85) -> (-14.325, -91.85)
  line L62 (-14.325, -91.85) -> (-28.325, -91.85)
  line L63 (-28.325, -91.85) -> (-28.325, -77.85)
  line L64 (-104.3, -91.85) -> (-104.3, -77.85)
  line L65 (-104.3, -77.85) -> (-90.3, -77.85)
  line L66 (-90.3, -77.85) -> (-90.3, -91.85)
  line L67 (-90.3, -91.85) -> (-104.3, -91.85)
  line L68 (-44.7, -95.65) -> (-44.7, -109.65)
  line L69 (-44.7, -109.65) -> (-58.7, -109.65)
  line L70 (-58.7, -109.65) -> (-58.7, -95.65)
  line L71 (-58.7, -95.65) -> (-44.7, -95.65)
  line L72 (-26.85, -95.65) -> (-26.85, -109.65)
  line L73 (-26.85, -109.65) -> (-40.85, -109.65)
  line L74 (-40.85, -109.65) -> (-40.85, -95.65)
  line L75 (-40.85, -95.65) -> (-26.85, -95.65)
  line L76 (-62.55, -95.65) -> (-62.55, -109.65)
  line L77 (-62.55, -109.65) -> (-76.55, -109.65)
  line L78 (-76.55, -109.65) -> (-76.55, -95.65)
  line L79 (-76.55, -95.65) -> (-62.55, -95.65)
  line L80 (-9, -95.65) -> (-9, -109.65)
  line L81 (-9, -109.65) -> (-23, -109.65)
  line L82 (-23, -109.65) -> (-23, -95.65)
  line L83 (-23, -95.65) -> (-9, -95.65)
  line L84 (-80.4, -95.65) -> (-80.4, -109.65)
  line L85 (-80.4, -109.65) -> (-94.4, -109.65)
  line L86 (-94.4, -109.65) -> (-94.4, -95.65)
  line L87 (-94.4, -95.65) -> (-80.4, -95.65)
  line L88 (-9, -113.5) -> (-9, -127.5)
  line L89 (-9, -127.5) -> (-23, -127.5)
  line L90 (-23, -127.5) -> (-23, -113.5)
  line L91 (-23, -113.5) -> (-9, -113.5)
  line L92 (0, -136.5) -> (0, -133)
  line L93 (0, -133) -> (-3.5, -133)
  circle A0 centre (-3.5, -133) radius 1.625
  dimension "d106" = 3.25
  constraint coincident L7 L92.end
  constraint parallel L7 L92
  constraint perpendicular L92 L93
  constraint coincident L93.end A0.centre
  measures "d106" diameter of A0
extrude "Extrude12" cut sketch "Sketch12" against normal blind 5 contours A0
sketch "Sketch13" plane through (0, 1.4, 0) normal (0, 1, 0) x (-1, 0, 0)
  circle A0 centre (-3.5, -133) radius 1.625
  line L0 (0, -38.25) -> (-124, -38.25)
  line L1 (-124, -38.25) -> (-124, -58)
  line L2 (-124, -58) -> (-102, -112)
  line L3 (-102, -112) -> (-96.5, -117.5)
  line L4 (-96.5, -117.5) -> (-25, -136.5)
  line L5 (-25, -136.5) -> (-2.5, -136.5)
  line L6 (-2.5, -136.5) -> (0, -134)
  line L7 (0, -134) -> (0, -38.25)
  line L8 (-68.85, -56.1) -> (-82.85, -56.1)
  line L9 (-82.85, -56.1) -> (-82.85, -42.1)
  line L10 (-82.85, -42.1) -> (-68.85, -42.1)
  line L11 (-68.85, -42.1) -> (-68.85, -56.1)
  line L12 (-51, -56.1) -> (-65, -56.1)
  line L13 (-65, -56.1) -> (-65, -42.1)
  line L14 (-65, -42.1) -> (-51, -42.1)
  line L15 (-51, -42.1) -> (-51, -56.1)
  line L16 (-86.7, -56.1) -> (-100.7, -56.1)
  line L17 (-100.7, -56.1) -> (-100.7, -42.1)
  line L18 (-100.7, -42.1) -> (-86.7, -42.1)
  line L19 (-86.7, -42.1) -> (-86.7, -56.1)
  line L20 (-21.075, -56.1) -> (-35.075, -56.1)
  line L21 (-35.075, -56.1) -> (-35.075, -42.1)
  line L22 (-35.075, -42.1) -> (-21.075, -42.1)
  line L23 (-21.075, -42.1) -> (-21.075, -56.1)
  line L24 (-104.55, -56.1) -> (-118.55, -56.1)
  line L25 (-118.55, -56.1) -> (-118.55, -42.1)
  line L26 (-118.55, -42.1) -> (-104.55, -42.1)
  line L27 (-104.55, -42.1) -> (-104.55, -56.1)
  line L28 (-62.7, -73.95) -> (-76.7, -73.95)
  line L29 (-76.7, -73.95) -> (-76.7, -59.95)
  line L30 (-76.7, -59.95) -> (-62.7, -59.95)
  line L31 (-62.7, -59.95) -> (-62.7, -73.95)
  line L32 (-44.85, -59.95) -> (-44.85, -73.95)
  line L33 (-44.85, -73.95) -> (-58.85, -73.95)
  line L34 (-58.85, -73.95) -> (-58.85, -59.95)
  line L35 (-58.85, -59.95) -> (-44.85, -59.95)
  line L36 (-80.55, -73.95) -> (-94.55, -73.95)
  line L37 (-94.55, -73.95) -> (-94.55, -59.95)
  line L38 (-94.55, -59.95) -> (-80.55, -59.95)
  line L39 (-80.55, -59.95) -> (-80.55, -73.95)
  line L40 (-19.675, -73.95) -> (-33.675, -73.95)
  line L41 (-33.675, -73.95) -> (-33.675, -59.95)
  line L42 (-33.675, -59.95) -> (-19.675, -59.95)
  line L43 (-19.675, -59.95) -> (-19.675, -73.95)
  line L44 (-98.4, -59.95) -> (-98.4, -73.95)
  line L45 (-98.4, -73.95) -> (-112.4, -73.95)
  line L46 (-112.4, -73.95) -> (-112.4, -59.95)
  line L47 (-112.4, -59.95) -> (-98.4, -59.95)
  line L48 (-68.6, -91.85) -> (-68.6, -77.85)
  line L49 (-68.6, -77.85) -> (-54.6, -77.85)
  line L50 (-54.6, -77.85) -> (-54.6, -91.85)
  line L51 (-54.6, -91.85) -> (-68.6, -91.85)
  line L52 (-50.75, -91.85) -> (-50.75, -77.85)
  line L53 (-50.75, -77.85) -> (-36.75, -77.85)
  line L54 (-36.75, -77.85) -> (-36.75, -91.85)
  line L55 (-36.75, -91.85) -> (-50.75, -91.85)
  line L56 (-86.45, -91.85) -> (-86.45, -77.85)
  line L57 (-86.45, -77.85) -> (-72.45, -77.85)
  line L58 (-72.45, -77.85) -> (-72.45, -91.85)
  line L59 (-72.45, -91.85) -> (-86.45, -91.85)
  line L60 (-28.325, -77.85) -> (-14.325, -77.85)
  line L61 (-14.325, -77.85) -> (-14.325, -91.85)
  line L62 (-14.325, -91.85) -> (-28.325, -91.85)
  line L63 (-28.325, -91.85) -> (-28.325, -77.85)
  line L64 (-104.3, -91.85) -> (-104.3, -77.85)
  line L65 (-104.3, -77.85) -> (-90.3, -77.85)
  line L66 (-90.3, -77.85) -> (-90.3, -91.85)
  line L67 (-90.3, -91.85) -> (-104.3, -91.85)
  line L68 (-44.7, -95.65) -> (-44.7, -109.65)
  line L69 (-44.7, -109.65) -> (-58.7, -109.65)
  line L70 (-58.7, -109.65) -> (-58.7, -95.65)
  line L71 (-58.7, -95.65) -> (-44.7, -95.65)
  line L72 (-26.85, -95.65) -> (-26.85, -109.65)
  line L73 (-26.85, -109.65) -> (-40.85, -109.65)
  line L74 (-40.85, -109.65) -> (-40.85, -95.65)
  line L75 (-40.85, -95.65) -> (-26.85, -95.65)
  line L76 (-62.55, -95.65) -> (-62.55, -109.65)
  line L77 (-62.55, -109.65) -> (-76.55, -109.65)
  line L78 (-76.55, -109.65) -> (-76.55, -95.65)
  line L79 (-76.55, -95.65) -> (-62.55, -95.65)
  line L80 (-9, -95.65) -> (-9, -109.65)
  line L81 (-9, -109.65) -> (-23, -109.65)
  line L82 (-23, -109.65) -> (-23, -95.65)
  line L83 (-23, -95.65) -> (-9, -95.65)
  line L84 (-80.4, -95.65) -> (-80.4, -109.65)
  line L85 (-80.4, -109.65) -> (-94.4, -109.65)
  line L86 (-94.4, -109.65) -> (-94.4, -95.65)
  line L87 (-94.4, -95.65) -> (-80.4, -95.65)
  line L88 (-9, -113.5) -> (-9, -127.5)
  line L89 (-9, -127.5) -> (-23, -127.5)
  line L90 (-23, -127.5) -> (-23, -113.5)
  line L91 (-23, -113.5) -> (-9, -113.5)
  line L92 (0, -136.5) -> (-36, -136.5)
  line L93 (-36, -136.5) -> (-36, -115)
  circle A1 centre (-36, -115) radius 1.625
  dimension "d109" = 36
  dimension "d110" = 21.5
  dimension "d111" = 3.25
  constraint parallel L5 L92
  constraint perpendicular L92 L93
  constraint coincident L93.end A1.centre
  measures "d109" distance of L92.start L92.end
  measures "d110" distance of L92.end L93.end
  measures "d111" diameter of A1
extrude "Extrude13" cut sketch "Sketch13" against normal blind 5 contours A1